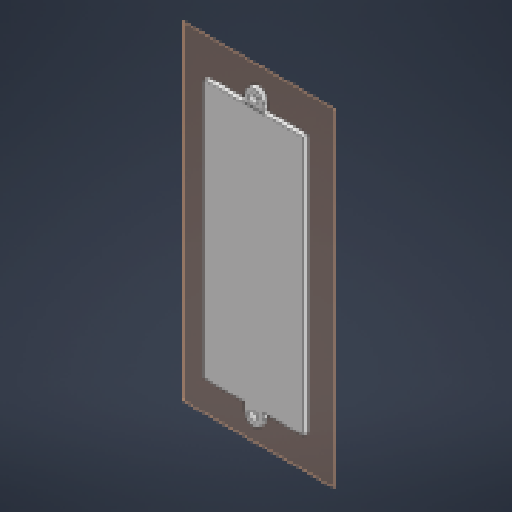
# Autodesk Inventor part: light fixture
Saved by Autodesk Inventor 2024.3 (Build 283343000, 343)
## iProperties
Created: 2025-08-06
Part Number: light fixture
Material: Generic
Document SubType Name: Modeling
Designer: giuseppe
Density: 1 g/cm^3
Appearance: Default
Author: giuseppe
Autodesk Inventor part; units mm, degrees
ref_plane "YZ Plane" through (0, 0, 0) normal (1, 0, 0) x (0, 1, 0)
ref_plane "XZ Plane" through (0, 0, 0) normal (0, 1, 0) x (-1, 0, 0)
ref_plane "XY Plane" through (0, 0, 0) normal (0, 0, 1) x (1, 0, 0)
ref_plane "Work Plane1" through (0, 0, 6) normal (0, 0, 1) x (1, 0, 0)
sketch "Sketch1" plane through (0, 0, 6) normal (0, 0, 1) x (1, 0, 0)
  line L0 (20.5, 53.1) -> (-20.5, 53.1) projected
  line L1 (-20.5, 53.1) -> (-20.5, -53.4) projected
  line L2 (-20.5, -53.4) -> (20.5, -53.4) projected
  line L3 (20.5, -53.4) -> (20.5, 53.1) projected
  line L4 (-18.5, 51.4) -> (-18.5, -51.4) projected
  line L5 (18.5, 51.4) -> (-18.5, 51.4) projected
  line L6 (18.5, -51.4) -> (18.5, 51.4) projected
  line L7 (-18.5, -51.4) -> (18.5, -51.4) projected
  point P0 (0, 0)
extrude "Extrusion1" add sketch "Sketch1" along normal blind 2 contours L3 L2 L1 L0 | L5 L6 L7 L4
sketch "Sketch2" plane through (0, 0, 8) normal (0, 0, 1) x (1, 0, 0)
  line L0 (-3.75, -53.4) -> (3.75, -53.4)
  line L1 (3.75, -53.4) -> (3.75, -56.4)
  line L2 (3.75, -56.4) -> (-3.75, -56.4)
  line L3 (-3.75, -56.4) -> (-3.75, -53.4)
  arc A0 (-3.75, -56.4) -> (3.75, -56.4) centre (0, -56.4) ccw
  circle A1 centre (0, -56.4) radius 1.75
  line L4 (-20.5, -53.4) -> (20.5, -53.4) projected
  point P0 (0, 0)
  dimension "d2" = 3.5
  dimension "d3" = 2
  dimension "d4" = 3
  constraints: 8 end point, 2 centre point, 2 parallel, 2 point on circle, 1 coincident, 1 collinear, 1 horizontal, 1 midpoint, 1 perpendicular, 1 vertical alignment
  measures "d2" diameter of A1
  measures "d3" radial gap between concentric circles of A0 A1
  measures "d4" distance of L2.end L0.start
extrude "Extrusion2" add sketch "Sketch2" against normal up to surface (2 mm away) contours L0 L1 L2 A1 L3 | L2 A1 A0
mirror "Mirror1" about plane through (0, 0, 0) normal (0, 1, 0) of "Extrusion2"
body "Solid1"
